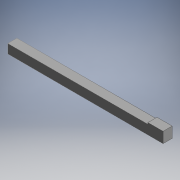
# Autodesk Inventor part: Whistle1
Saved by Autodesk Inventor 2018 (Build 220112000, 112)
## iProperties
Created: 2018-09-27
Part Number: Whistle1
Material: Generic
Document SubType Name: Modeling
Designer: Isaac Newcomb
Density: 1 g/cm^3
Appearance: Default
MaxWidth: 10.000 mm
PlugLength: 20.000 mm
Author: Isaac Newcomb
Autodesk Inventor part; units mm, degrees
ref_plane "YZ Plane" through (0, 0, 0) normal (1, 0, 0) x (0, 1, 0)
ref_plane "XZ Plane" through (0, 0, 0) normal (0, 1, 0) x (-1, 0, 0)
ref_plane "XY Plane" through (0, 0, 0) normal (0, 0, 1) x (1, 0, 0)
sketch "Tube Base Sketch" plane through (0, 0, 0) normal (0, 0, 1) x (1, 0, 0)
  line L0 (-5, -5) -> (5, -5)
  line L1 (5, -5) -> (5, 5)
  line L2 (5, 5) -> (-5, 5)
  line L3 (-5, 5) -> (-5, -5)
  line L4 (-5, -5) -> (5, 5) construction
  line L5 (5, -5) -> (-5, 5) construction
  line L6 (-6, 6) -> (6, 6)
  line L7 (6, 6) -> (6, -6)
  line L8 (6, -6) -> (-6, -6)
  line L9 (-6, -6) -> (-6, 6)
  point P0 (0, 0)
  dimension "d16" = 10
  dimension "d17" = 10
  dimension "WallThickness" = 1
  constraints: 20 end point, 4 parallel, 2 midpoint, 2 perpendicular, 1 horizontal, 3 other
  measures "d16" distance of L2.end L1.end
  measures "d17" distance of L1.end L0.end
  measures "WallThickness" distance between parallel lines of L2 L6
extrude "Tube" add sketch "Tube Base Sketch" along normal blind 184.2137
sketch "Cap Sketch" plane through (0, 0, 0) normal (0, 0, -1) x (-1, 0, 0)
  line L0 (-6, -6) -> (6, -6)
  line L1 (6, -6) -> (6, 8)
  line L2 (6, 8) -> (-6, 8)
  line L3 (-6, 8) -> (-6, -6)
  point P0 (0, 0)
  dimension "CapHeight" = 14
  constraints: 8 end point, 2 parallel, 1 coincident, 1 horizontal, 1 perpendicular
  measures "CapHeight" distance of L1.end L0.end
extrude "Extrusion6" add sketch "Cap Sketch" along normal blind 20
equation "\"d16\" = MaxWidth"
equation "\"d17\" = MaxWidth"
equation "\"TubeLength\" = DesiredLength + PlugLength"
equation "\"MaxWidth\" = 10"
equation "\"DesiredLength\" = 164.21369"
equation "\"PlugLength\" = 20"
body "Solid2"
